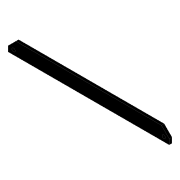
# Autodesk Inventor part: road
Saved by Autodesk Inventor 2020 (Build 240168000, 168)
## iProperties
Created: 2021-07-09
Part Number: road
Material: Generic
Document SubType Name: Modeling
Designer: Aidan Lee
Density: 1 g/cm^3
Appearance: Anodized - Black
Author: Aidan Lee
Autodesk Inventor part; units mm, degrees
ref_plane "YZ Plane" through (0, 0, 0) normal (1, 0, 0) x (0, 1, 0)
ref_plane "XZ Plane" through (0, 0, 0) normal (0, 1, 0) x (-1, 0, 0)
ref_plane "XY Plane" through (0, 0, 0) normal (0, 0, 1) x (1, 0, 0)
sketch "Sketch1" plane through (0, 0, 0) normal (0, 0, 1) x (1, 0, 0)
  line L0 (0, 0) -> (0, 9.712)
  line L1 (0, 9.712) -> (14.5, 24.212)
  line L2 (14.5, 24.212) -> (149.675, 24.212)
  line L3 (0, 0) -> (149.675, 0)
  circle A0 centre (10.1, 8) radius 3
  line L4 (149.675, 42.0637) -> (149.675, 59.6175)
  line L5 (299.35, 0) -> (299.35, 9.712)
  line L6 (299.35, 9.712) -> (284.85, 24.212)
  line L7 (284.85, 24.212) -> (149.675, 24.212)
  line L8 (299.35, 0) -> (149.675, 0)
  circle A1 centre (289.25, 8) radius 3
  dimension "d0" = 135
  dimension "d1" = 149.675
  dimension "d2" = 9.712
  dimension "d3" = 24.212
  dimension "d4" = 6
  dimension "d5" = 8
  dimension "d6" = 10.1
  constraints: 18 end point, 4 symmetric about line, 2 centre point, 2 vertical, 2 vertical alignment, 1 horizontal, 1 perpendicular, 1 other
  measures "d0" angle of L0 L1
  measures "d1" distance of L0.start L3.end
  measures "d2" distance of L0.start L0.end
  measures "d3" distance between parallel lines of L3 L2
  measures "d4" diameter of A0
  measures "d5" distance from line of L3 A0.centre
  measures "d6" distance from line of A0.centre L0
extrude "Extrusion1" add sketch "Sketch1" along normal blind 5
body "Solid1"
